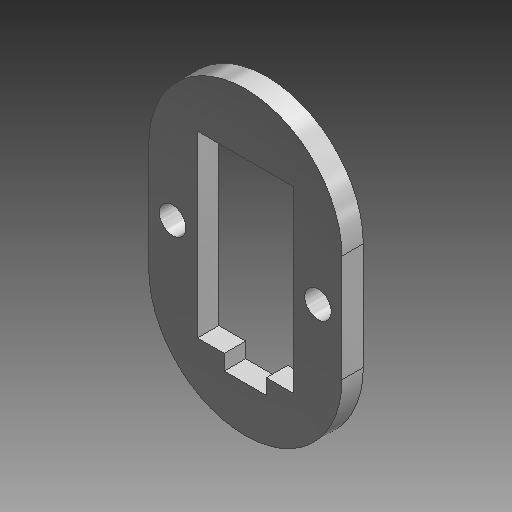
# Autodesk Inventor part: Part1
Saved by Autodesk Inventor 2019.2 (Build 232265000, 265)
## iProperties
Part Number: Part1
Material: LCP Plastic
Document SubType Name: Modeling
Designer: richard.girt
Mass: 2.4198 g
Surface Area: 16.3732 cm^2
Volume: 1.48819 cm^3
Density: 1.626 g/cm^3
Appearance: Smooth - White
Author: richard.girt
Autodesk Inventor part; units mm, degrees
ref_plane "YZ Plane" through (0, 0, 0) normal (1, 0, 0) x (0, 1, 0)
ref_plane "XZ Plane" through (0, 0, 0) normal (0, 1, 0) x (-1, 0, 0)
ref_plane "XY Plane" through (0, 0, 0) normal (0, 0, 1) x (1, 0, 0)
sketch "Sketch1" plane through (0, 0, 0) normal (0, 0, 1) x (1, 0, 0)
  line L0 (0, -7) -> (0, 7) construction
  line L1 (12.625, -7) -> (12.625, 7)
  line L2 (-12.625, 7) -> (-12.625, -7)
  arc A0 (-12.625, -7) -> (12.625, -7) centre (0, -7) ccw
  arc A1 (12.625, 7) -> (-12.625, 7) centre (0, 7) ccw
  circle A2 centre (0, 0) radius 9.5 construction
  circle A3 centre (-9.5, 0) radius 1.75
  circle A4 centre (9.5, 0) radius 1.75
  line L3 (-6.25, -11.7) -> (6.25, -11.7)
  line L4 (6.25, -11.7) -> (6.25, 11.7)
  line L5 (6.25, 11.7) -> (-6.25, 11.7)
  line L6 (-6.25, 11.7) -> (-6.25, -11.7)
  line L7 (-6.25, -11.7) -> (6.25, 11.7) construction
  line L8 (6.25, -11.7) -> (-6.25, 11.7) construction
  line L9 (-2.75, -13.7) -> (2.75, -13.7)
  line L10 (2.75, -13.7) -> (2.75, -11.7)
  line L11 (2.75, -11.7) -> (-2.75, -11.7)
  line L12 (-2.75, -11.7) -> (-2.75, -13.7)
  point P0 (0, -11.7)
  dimension "d2" = 14
  dimension "d3" = 12.625
  dimension "d4" = 19
  dimension "d5" = 3.5
  dimension "d6" = 12.5
  dimension "d7" = 23.4
  dimension "d8" = 5.5
  dimension "d9" = 2
  constraints: 28 end point, 6 point on circle, 5 centre point, 5 midpoint, 5 parallel, 4 tangent, 2 horizontal, 2 horizontal alignment, 2 perpendicular, 1 coincident, 1 equal radius, 1 vertical
  measures "d2" distance of L0.start L0.end
  measures "d3" radius of A0
  measures "d4" diameter of A2
  measures "d5" diameter of A3
  measures "d6" distance of L4.end L5.end
  measures "d7" distance of L3.end L4.end
  measures "d8" distance of L9.start L9.end
  measures "d9" distance of L11.end L9.start
extrude "Extrusion1" add sketch "Sketch1" against normal blind 2.8
body "Solid1"
